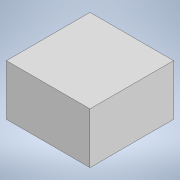
# Autodesk Inventor part: Aluminium block mold
Saved by Autodesk Inventor 2020 (Build 240168000, 168)
## iProperties
Created: 2022-08-29
Part Number: Aluminium block mold
Material: Generic
Document SubType Name: Modeling
Designer: Administrator
Density: 1 g/cm^3
Appearance: Default
Author: Administrator
Autodesk Inventor part; units mm, degrees
ref_plane "YZ Plane" through (0, 0, 0) normal (1, 0, 0) x (0, 1, 0)
ref_plane "XZ Plane" through (0, 0, 0) normal (0, 1, 0) x (-1, 0, 0)
ref_plane "XY Plane" through (0, 0, 0) normal (0, 0, 1) x (1, 0, 0)
sketch "Sketch1" plane through (0, 0, 0) normal (0, 1, 0) x (-1, 0, 0)
  line L0 (45, -45) -> (-45, -45)
  line L1 (-45, -45) -> (-45, 45)
  line L2 (-45, 45) -> (45, 45)
  line L3 (45, 45) -> (45, -45)
  line L4 (45, -45) -> (-45, 45) construction
  line L5 (-45, -45) -> (45, 45) construction
  line L6 (-46, -46) -> (46, -46)
  line L7 (46, -46) -> (46, 46)
  line L8 (46, 46) -> (-46, 46)
  line L9 (-46, 46) -> (-46, -46)
  line L10 (-46, -46) -> (46, 46) construction
  line L11 (46, -46) -> (-46, 46) construction
  point P0 (0, 0)
  dimension "d0" = 90
  dimension "d1" = 90
  dimension "d4" = 92
  dimension "d5" = 92
  constraints: 24 end point, 4 midpoint, 4 parallel, 2 horizontal, 2 perpendicular
  measures "d0" distance of L1.end L2.end
  measures "d1" distance of L0.end L1.end
  measures "d4" distance of L8.end L7.end
  measures "d5" distance of L7.end L6.end
extrude "Extrusion1" add sketch "Sketch1" along normal blind 55
sketch "Sketch2" plane through (0, 55, 0) normal (0, 1, 0) x (1, 0, 0)
  line L0 (-46, 46) -> (-46, -46) projected
  line L1 (46, 46) -> (-46, 46)
  line L2 (-46, 46) -> (-46, -46)
  line L3 (-46, -46) -> (46, -46)
  line L4 (46, -46) -> (46, 46)
  line L5 (46, 46) -> (-46, -46) construction
  line L6 (-46, 46) -> (46, -46) construction
  point P0 (0, 0)
  constraints: 12 end point, 2 midpoint, 2 parallel, 1 horizontal, 1 perpendicular
extrude "Extrusion2" add sketch "Sketch2" along normal blind 1
body "Solid1"
